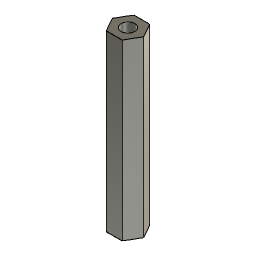
M3_Standoff v1 (Autodesk Fusion 360 design; units mm, degrees)
Autodesk Fusion 360 part; units mm, degrees
sketch "Sketch1" plane through (0, 0, 0) normal (0, 0, 1) x (1, 0, 0)
  line L0 (1.7321, -3) -> (3.4641, 0)
  line L1 (3.4641, 0) -> (1.7321, 3)
  line L2 (1.7321, 3) -> (-1.7321, 3)
  line L3 (-1.7321, 3) -> (-3.4641, 0)
  line L4 (-3.4641, 0) -> (-1.7321, -3)
  line L5 (-1.7321, -3) -> (1.7321, -3)
  circle A0 centre (0, 0) radius 1.5
  dimension "d1" = 3
  dimension "d2" = 3
  constraint coincident A0.centre origin
  measures "d1" distance of A0.centre L5
  measures "d2" diameter of A0
extrude "Extrude1" add sketch "Sketch1" along normal blind 38
